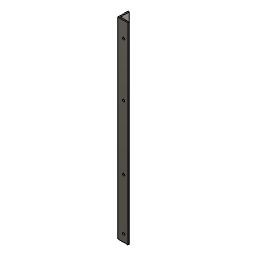
angle iron 1 inch 480 mm Opposite v1 (Autodesk Fusion 360 design; units mm, degrees)
Autodesk Fusion 360 part; units mm, degrees
sketch "Sketch1" plane through (0, 0, 0) normal (0, 1, 0) x (1, 0, 0)
  line L0 (0, 0) -> (25.4, 0)
  line L1 (25.4, 0) -> (25.4, -3.175)
  line L2 (25.4, -3.175) -> (3.175, -3.175)
  line L3 (3.175, -3.175) -> (3.175, -25.4)
  line L4 (3.175, -25.4) -> (0, -25.4)
  line L5 (0, -25.4) -> (0, 0)
  dimension "d1" = 25.4
  dimension "d2" = 25.4
  dimension "d3" = 3.175
  dimension "d4" = 3.175
  constraint coincident L0.start L5.end
  constraint horizontal L0
  constraint perpendicular L0 L1
  constraint perpendicular L1 L2
  constraint perpendicular L0 L3
  constraint perpendicular L3 L4
  constraint perpendicular L0 L5
  measures "d1" distance of L0.start L0.end
  measures "d2" distance of L4.end L0.start
  measures "d3" distance of L3 L5
  measures "d4" distance of L0 L2
extrude "Extrude1" add sketch "Sketch1" along normal blind 480 makes body 1
sketch "Sketch2" plane through (0, 0, 3.175) normal (0, 0, 1) x (1, 0, 0)
  line L0 (3.175, 0) -> (25.4, 0)
  line L1 (25.4, 0) -> (25.4, 480)
  line L2 (25.4, 480) -> (3.175, 480)
  line L3 (3.175, 480) -> (3.175, 0)
  circle A0 centre (14.2875, 18.25) radius 2.75
  circle A1 centre (14.2875, 146.11) radius 2.75
  circle A2 centre (14.2875, 306.51) radius 2.75
  circle A3 centre (14.2875, 440.31) radius 2.75
  line L4 (14.2875, 480) -> (14.2875, 0) construction
  dimension "d7" = 18.25
  dimension "d8" = 146.11
  dimension "d9" = 306.51
  dimension "d10" = 440.31
  dimension "d11" = 5.5
  constraint equal A2 A3
  constraint equal A1 A2
  constraint equal A0 A1
  constraint midpoint L2 L4.start
  constraint midpoint L0 L4.end
  constraint coincident A0.centre L4
  constraint coincident A1.centre L4
  constraint coincident A2.centre L4
  constraint coincident A3.centre L4
  measures "d7" distance of L0 A0.centre
  measures "d8" distance of L0 A1.centre
  measures "d9" distance of L0 A2.centre
  measures "d10" distance of L0 A3.centre
  measures "d11" diameter of A1
sketch "Sketch3" plane through (3.175, 0, 0) normal (1, 0, 0) x (0, 0, -1)
  line L0 (-25.4, 0) -> (-3.175, 0)
  line L1 (-3.175, 0) -> (-3.175, 480)
  line L2 (-3.175, 480) -> (-25.4, 480)
  line L3 (-25.4, 480) -> (-25.4, 0)
  circle A0 centre (-14.2875, 120.71) radius 2.75
  circle A1 centre (-14.2875, 281.11) radius 2.75
  circle A2 centre (-14.2875, 465.71) radius 2.75
  line L4 (-14.2875, 480) -> (-14.2875, 0) construction
  dimension "d12" = 120.71
  dimension "d13" = 5.5
  dimension "d14" = 281.11
  dimension "d15" = 465.71
  constraint equal A1 A2
  constraint equal A0 A1
  constraint midpoint L2 L4.start
  constraint midpoint L0 L4.end
  constraint coincident A2.centre L4
  constraint coincident A1.centre L4
  constraint coincident A0.centre L4
  measures "d12" distance of L0 A0.centre
  measures "d13" diameter of A2
  measures "d14" distance of L0 A1.centre
  measures "d15" distance of L0 A2.centre
hole "Hole1" at (3.175, 465.71, 14.2875) at (3.175, 281.11, 14.2875) at (3.175, 120.71, 14.2875) direction (-1, 0, 0) diameter 5.5 depth 7 tip angle 118 bodies 1
hole "Hole2" at (14.2875, 440.31, 3.175) at (14.2875, 306.51, 3.175) at (14.2875, 146.11, 3.175) at (14.2875, 18.25, 3.175) direction (0, 0, -1) diameter 5.5 depth 7 tip angle 118 bodies 1
mirror "Mirror1" about plane through (0, 0, 0) normal (0, 0, 1) of bodies 1 merged
split "Split1" by plane through (0, 0, 0) normal (0, 0, 1) bodies 1 makes body 2 at (0, 39.3339, 13.07)
hidden bodies 2
equation "d3 = ( 1 / 8 ) * 1 in"
equation "d4 = ( 1 / 8 ) * 1 in"
equation "d8 = 135 mm + 11.11 mm"
equation "d9 = 295.4 mm + 11.11 mm"
equation "d10 = 429.2 mm + 11.11 mm"
equation "d12 = 109.6 mm + 11.11 mm"
equation "d14 = 270 mm + 11.11 mm"
equation "d15 = 454.6 mm + 11.11 mm"
